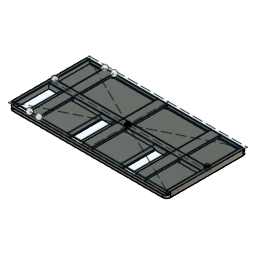
Center Cover 1x3 v4 (Autodesk Fusion 360 design; units mm, degrees)
Autodesk Fusion 360 part; units mm, degrees
sketch "Schizzo1" plane through (0, 0, 0) normal (0, 0, 1) x (1, 0, 0)
  line L0 (50, 150) -> (168.7, 150) construction
  line L1 (168.7, 150) -> (168.7, 89.3) construction
  line L2 (168.7, 89.3) -> (50, 89.3) construction
  line L3 (50, 89.3) -> (50, 150) construction
  line L4 (50, 119.65) -> (168.7, 119.65) construction
  line L5 (109.35, 150) -> (109.35, 89.3) construction
  line L6 (168.6, 89.4) -> (50.1, 89.4)
  line L7 (50.1, 89.4) -> (50.1, 149.9)
  line L8 (50.1, 149.9) -> (168.6, 149.9)
  line L9 (168.6, 149.9) -> (168.6, 89.4)
  line L10 (168.6, 89.4) -> (50.1, 149.9) construction
  line L11 (50.1, 89.4) -> (168.6, 149.9) construction
  point P0 (109.35, 119.65)
  dimension "d1" = 118.7
  dimension "d2" = 60.7
  dimension "d3" = 0.1
  dimension "d4" = 0.1
  constraint horizontal L0
  constraint vertical L1
  constraint horizontal L2
  constraint vertical L3
  constraint midpoint L3 L4.start
  constraint midpoint L1 L4.end
  constraint midpoint L0 L5.start
  constraint midpoint L2 L5.end
  constraint horizontal L6
  constraint perpendicular L6 L7
  constraint parallel L6 L8
  constraint parallel L7 L9
  constraint coincident L10 P0
  constraint coincident L11 P0
  constraint midpoint L4 P0
  measures "d1" distance of L0.start L0.end
  measures "d2" distance of L0 L2
  measures "d3" distance of L3 L7
  measures "d4" distance of L0 L8
extrude "Estrusione1" add sketch "Schizzo1" along normal blind 4
fillet "Raccordo1" radius 3 4 edges at (50.1, 89.4, 2) (168.6, 89.4, 2) (50.1, 149.9, 2) (168.6, 149.9, 2)
sketch "Schizzo2" plane through (0, 0, 4) normal (0, 0, 1) x (-1, 0, 0)
  arc A0 (-168.6, -146.9) -> (-165.6, -149.9) centre (-165.6, -146.9) ccw
  line L0 (-165.6, -149.9) -> (-53.1, -149.9)
  arc A1 (-53.1, -149.9) -> (-50.1, -146.9) centre (-53.1, -146.9) ccw
  line L1 (-50.1, -146.9) -> (-50.1, -92.4)
  arc A2 (-50.1, -92.4) -> (-53.1, -89.4) centre (-53.1, -92.4) ccw
  line L2 (-53.1, -89.4) -> (-165.6, -89.4)
  arc A3 (-165.6, -89.4) -> (-168.6, -92.4) centre (-165.6, -92.4) ccw
  line L3 (-168.6, -92.4) -> (-168.6, -146.9)
  line L4 (-50.1, -149.9) -> (-168.6, -149.9) construction
  line L5 (-168.6, -149.9) -> (-168.6, -89.4) construction
  line L6 (-168.6, -89.4) -> (-50.1, -89.4) construction
  line L7 (-50.1, -89.4) -> (-50.1, -149.9) construction
  line L8 (-50.1, -119.65) -> (-168.6, -119.65) construction
  line L9 (-109.35, -149.9) -> (-109.35, -89.4) construction
  line L10 (-166.6, -91.4) -> (-52.1, -91.4)
  line L11 (-52.1, -91.4) -> (-52.1, -147.9)
  line L12 (-52.1, -147.9) -> (-166.6, -147.9)
  line L13 (-166.6, -147.9) -> (-166.6, -91.4)
  line L14 (-166.6, -91.4) -> (-52.1, -147.9) construction
  line L15 (-52.1, -91.4) -> (-166.6, -147.9) construction
  line L16 (-70.6, -91.4) -> (-70.6, -147.9)
  line L17 (-63.6, -147.9) -> (-63.6, -91.4)
  line L18 (-52.1, -121.9) -> (-52.1, -147.9)
  line L19 (-103.6, -147.9) -> (-103.6, -91.4)
  line L20 (-110.6, -147.9) -> (-110.6, -91.4)
  line L21 (-143.6, -147.9) -> (-143.6, -91.4)
  line L22 (-150.6, -147.9) -> (-150.6, -91.4)
  line L23 (-52.1, -91.4) -> (-62.1, -91.4)
  line L24 (-62.1, -91.4) -> (-62.1, -117.4)
  line L25 (-62.1, -117.4) -> (-52.1, -117.4)
  line L26 (-52.1, -117.4) -> (-52.1, -91.4)
  line L27 (-102.1, -117.4) -> (-92.1, -117.4)
  line L28 (-92.1, -117.4) -> (-92.1, -91.4)
  line L29 (-102.1, -91.4) -> (-102.1, -117.4)
  line L30 (-92.1, -91.4) -> (-102.1, -91.4)
  line L31 (-142.1, -117.4) -> (-132.1, -117.4)
  line L32 (-132.1, -117.4) -> (-132.1, -91.4)
  line L33 (-142.1, -91.4) -> (-142.1, -117.4)
  line L34 (-132.1, -91.4) -> (-142.1, -91.4)
  line L35 (-52.1, -117.4) -> (-166.6, -117.4)
  line L36 (-52.1, -121.9) -> (-166.6, -121.9)
  point P0 (-109.35, -119.65)
  point P1 (-109.35, -119.65)
  dimension "d11" = 7
  dimension "d20" = 7
  dimension "d25" = 7
  dimension "d36" = 13.5
  dimension "d37" = 53.5
  dimension "d38" = 93.5
  dimension "d39" = 10
  dimension "d40" = 26
  dimension "d41" = 2
  dimension "d42" = 2
  dimension "d45" = -40
  dimension "d46" = 0
  constraint horizontal L4
  constraint vertical L5
  constraint horizontal L6
  constraint vertical L7
  constraint collinear L0 L4
  constraint collinear L1 L7
  constraint collinear L2 L6
  constraint collinear L3 L5
  constraint midpoint L7 L8.start
  constraint midpoint L5 L8.end
  constraint midpoint L4 L9.start
  constraint midpoint L6 L9.end
  constraint horizontal L10
  constraint perpendicular L10 L11
  constraint parallel L10 L12
  constraint parallel L11 L13
  constraint coincident L14 P1
  constraint coincident L15 P1
  constraint midpoint L9 P1
  constraint parallel L16 L17
  constraint coincident P1 P0
  constraint vertical L18
  constraint coincident L11.end L12.start
  constraint coincident L12 L19.start
  constraint coincident L10 L19.end
  constraint perpendicular L10 L19
  constraint coincident L12 L20.start
  constraint coincident L10 L20.end
  constraint perpendicular L10 L20
  constraint coincident L12 L21.start
  constraint coincident L10 L21.end
  constraint perpendicular L10 L21
  constraint coincident L12 L22.start
  constraint coincident L10 L22.end
  constraint perpendicular L10 L22
  constraint horizontal L23
  constraint vertical L24
  constraint horizontal L25
  constraint vertical L26
  constraint coincident L13 L35.end
  constraint perpendicular L13 L35
  constraint symmetric L8 L25.end L18.start
  constraint symmetric L8 L35.end L36.end
  measures "d11" distance of L16.end L17.start
  measures "d20" distance of L19 L20
  measures "d25" distance of L21 L22
  measures "d36" distance of L7 L17
  measures "d37" distance of L7 L19
  measures "d38" distance of L7 L21
  measures "d39" distance of L10.end L23.end
  measures "d40" distance of L10.end L25.end
  measures "d41" distance of L4 L12
  measures "d42" distance of L7 L11
extrude "Estrusione2" cut sketch "Schizzo2" against normal blind 3 contours L10 L13 L22 L35 | L10 L21 L33 L35 | L12 L13 L22 L36 | L10 L31 L32 L33 L34 L35 | L10 L20 L32 L35 | L12 L20 L21 L36 | L10 L19 L29 L35 | L12 L16 L19 L36 | L10 L27 L28 L29 L30 L35 | L10 L16 L28 L35 | L11 L12 L17 L18 L36 | L10 L17 L24 L35 | L10 L11 L23 L24 L25 L26 L35
extrude "Estrusione3" cut sketch "Schizzo2" against normal blind 4 contours L10 L31 L32 L33 L34 L35 | L10 L27 L28 L29 L30 L35 | L10 L11 L23 L24 L25 L26 L35
ref_plane "Piano di lavoro1" through (109.35, 119.65, 4) normal (0, -1, 0) x (1, 0, 0)
sketch "Schizzo3" plane through (0, 119.65, 0) normal (0, -1, 0) x (-1, 0, 0)
  line L0 (-50.1, -4) -> (-168.7, -4) construction
  line L1 (-168.7, -4) -> (-168.7, 0) construction
  line L2 (-168.7, 0) -> (-50.1, 0) construction
  line L3 (-50.1, 0) -> (-50.1, -4) construction
  line L4 (-168.6, -4) -> (-50.1, -4) construction
  line L5 (-50.1, -1) -> (-168.7, -1) construction
  line L6 (-63.6, -4) -> (-63.6, 0) construction
  line L7 (-70.6, -4) -> (-70.6, 0) construction
  line L8 (-63.6, -4) -> (-63.6, -1) construction
  line L9 (-70.6, -4) -> (-70.6, -1) construction
  line L10 (-103.6, -4) -> (-103.6, 0) construction
  line L11 (-110.6, -4) -> (-110.6, 0) construction
  line L12 (-103.6, -4) -> (-103.6, -1) construction
  line L13 (-110.6, -4) -> (-110.6, -1) construction
  line L14 (-143.6, -4) -> (-143.6, 0) construction
  line L15 (-150.6, -4) -> (-150.6, 0) construction
  line L16 (-143.6, -4) -> (-143.6, -1) construction
  line L17 (-150.6, -4) -> (-150.6, -1) construction
  line L18 (-63.6, -4) -> (-65.3321, -1)
  line L19 (-63.6, -4) -> (-60.1359, -4) construction
  line L20 (-70.6, -4) -> (-68.8679, -1)
  line L21 (-70.6, -4) -> (-67.1359, -4) construction
  line L22 (-63.6, -4) -> (-63.6, -1)
  line L23 (-63.6, -1) -> (-65.3321, -1)
  line L24 (-68.8679, -1) -> (-70.6, -1)
  line L25 (-70.6, -1) -> (-70.6, -4)
  line L26 (-103.6, -1) -> (-103.6, -4)
  line L27 (-103.6, -4) -> (-105.3321, -1)
  line L28 (-105.3321, -1) -> (-103.6, -1)
  line L29 (-110.6, -1) -> (-110.6, -4)
  line L30 (-110.6, -4) -> (-108.8679, -1)
  line L31 (-108.8679, -1) -> (-110.6, -1)
  line L32 (-143.6, -1) -> (-143.6, -4)
  line L33 (-143.6, -4) -> (-145.3321, -1)
  line L34 (-145.3321, -1) -> (-143.6, -1)
  line L35 (-150.6, -1) -> (-150.6, -4)
  line L36 (-150.6, -4) -> (-148.8679, -1)
  line L37 (-148.8679, -1) -> (-150.6, -1)
  line L38 (-110.6, -1) -> (-143.6, -1)
  point P0 (-168.7, 0)
  dimension "d28" = 120
  dimension "d29" = 60
  dimension "d30" = 30
  dimension "d31" = 30
  dimension "d32" = 30
  dimension "d33" = 30
  constraint horizontal L0
  constraint vertical L1
  constraint horizontal L2
  constraint vertical L3
  constraint coincident L0.start L3.end
  constraint coincident P0 L1.end
  constraint coincident L3 L5.start
  constraint coincident L1 L5.end
  constraint perpendicular L1 L5
  constraint coincident L4 L6.start
  constraint coincident L2 L6.end
  constraint perpendicular L2 L6
  constraint coincident L0 L7.start
  constraint coincident L2 L7.end
  constraint perpendicular L2 L7
  constraint collinear L6 L8
  constraint collinear L7 L9
  constraint coincident L0 L10.start
  constraint coincident L2 L10.end
  constraint perpendicular L2 L10
  constraint coincident L0 L11.start
  constraint coincident L2 L11.end
  constraint perpendicular L2 L11
  constraint collinear L10 L12
  constraint collinear L11 L13
  constraint coincident L0 L14.start
  constraint coincident L2 L14.end
  constraint perpendicular L2 L14
  constraint coincident L0 L15.start
  constraint coincident L2 L15.end
  constraint perpendicular L2 L15
  constraint collinear L14 L16
  constraint collinear L15 L17
  constraint horizontal L19
  constraint coincident L5 L18.end
  constraint horizontal L21
  constraint coincident L7.start L9.start
  constraint coincident L5 L20.end
  constraint coincident L8.end L22.end
  constraint coincident L9.end L24.end
  constraint coincident L12.end L26.start
  constraint coincident L10.start L12.start
  constraint coincident L5 L27.end
  constraint coincident L11.start L13.start
  constraint coincident L5 L30.end
  constraint coincident L16.end L32.start
  constraint coincident L14.start L16.start
  constraint coincident L5 L33.end
  constraint coincident L17.end L35.start
  constraint coincident L15.start L17.start
  constraint coincident L5 L36.end
  constraint coincident L13.end L38
  constraint coincident L5 L13.end
  constraint parallel L31 L38
  constraint vertical L29
  measures "d28" angle of L18 L19
  measures "d29" angle of L20 L21
  measures "d30" angle of L26 L27
  measures "d31" angle of L29 L30
  measures "d32" angle of L32 L33
  measures "d33" angle of L35 L36
extrude "Estrusione4" cut sketch "Schizzo3" along normal blind 25 from surface at 2.5
extrude "Estrusione6" cut sketch "Schizzo3" against normal blind 25 from surface at -2.5
sketch "Schizzo4" plane through (0, 0, 4) normal (0, 0, 1) x (-1, 0, 0)
  line L0 (-50.1, -149.9) -> (-168.6, -149.9) construction
  line L1 (-168.6, -149.9) -> (-168.6, -89.4) construction
  line L2 (-168.6, -89.4) -> (-50.1, -89.4) construction
  line L3 (-50.1, -89.4) -> (-50.1, -149.9) construction
  line L4 (-165.6, -149.9) -> (-53.1, -149.9) construction
  line L5 (-53.1, -89.4) -> (-165.6, -89.4) construction
  line L6 (-50.1, -146.9) -> (-50.1, -92.4) construction
  line L7 (-168.6, -92.4) -> (-168.6, -146.9) construction
  line L8 (-50.1, -149.9) -> (-168.6, -149.9)
  line L9 (-168.6, -149.9) -> (-168.6, -147.9)
  line L10 (-168.6, -147.9) -> (-50.1, -147.9)
  line L11 (-50.1, -147.9) -> (-50.1, -149.9)
  line L12 (-50.1, -89.4) -> (-168.6, -89.4)
  line L13 (-168.6, -89.4) -> (-168.6, -91.4)
  line L14 (-168.6, -91.4) -> (-50.1, -91.4)
  line L15 (-50.1, -91.4) -> (-50.1, -89.4)
  dimension "d51" = 2
  dimension "d52" = 2
  constraint horizontal L0
  constraint vertical L1
  constraint horizontal L2
  constraint vertical L3
  constraint collinear L0 L4
  constraint collinear L2 L5
  constraint collinear L3 L6
  constraint collinear L1 L7
  constraint horizontal L8
  constraint vertical L9
  constraint horizontal L10
  constraint vertical L11
  constraint horizontal L12
  constraint vertical L13
  constraint horizontal L14
  constraint vertical L15
  measures "d51" distance of L0.start L10.end
  measures "d52" distance of L2.end L14.end
extrude "Estrusione5" cut sketch "Schizzo4" against normal blind 2
equation "d28 = 90 deg + 30 deg"
equation "d52 = d51"
